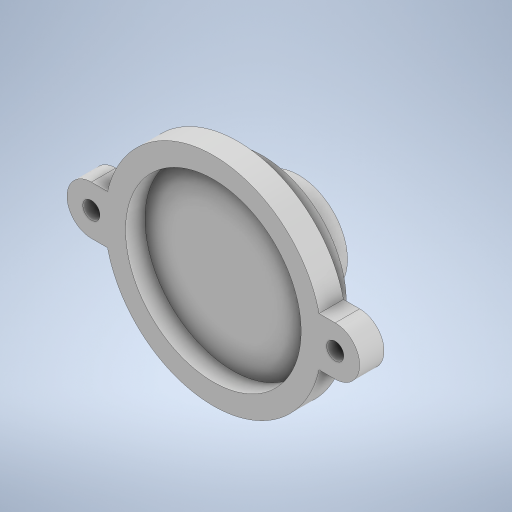
# Autodesk Inventor part: Prato do Amassador
Saved by Autodesk Inventor 2023 (Build 270158030, 158C)
## iProperties
Created: 2022-07-18
Part Number: Prato do Amassador
Material: Generic
Document SubType Name: Modeling
Designer: coqui
Density: 1 g/cm^3
Appearance: Default
Author: coqui
Autodesk Inventor part; units mm, degrees
ref_plane "YZ Plane" through (0, 0, 0) normal (1, 0, 0) x (0, 1, 0)
ref_plane "XZ Plane" through (0, 0, 0) normal (0, 1, 0) x (-1, 0, 0)
ref_plane "XY Plane" through (0, 0, 0) normal (0, 0, 1) x (1, 0, 0)
sketch "Sketch1" plane through (0, 0, 0) normal (0, 0, 1) x (1, 0, 0)
  arc A0 (50, -10) -> (50, 10) centre (50, 0) ccw
  arc A1 (-50, 10) -> (-50, -10) centre (-50, 0) ccw
  arc A2 (-43.3618, -10) -> (43.3618, -10) centre (0, 0) ccw
  arc A3 (43.3618, 10) -> (-43.3618, 10) centre (0, 0) ccw
  circle A4 centre (-50, 0) radius 3.5
  circle A5 centre (50, 0) radius 3.5
  line L0 (50, -10) -> (43.3618, -10)
  line L1 (-43.3618, -10) -> (-50, -10)
  line L2 (-50, 10) -> (-43.3618, 10)
  line L3 (43.3618, 10) -> (50, 10)
  dimension "d1" = 20
  dimension "d2" = 20
  dimension "d4" = 50
  dimension "d5" = 50
  dimension "d6" = 7
  dimension "d7" = 7
  constraints: 8 end point, 8 point on circle, 6 centre point, 6 tangent, 3 coincident
  measures "d1" diameter of A0
  measures "d2" diameter of A1
  measures "d4" distance of A0.centre point (0, 0)
  measures "d5" distance of point (0, 0) A1.centre
  measures "d6" diameter of A4
  measures "d7" diameter of A5
extrude "Extrusion1" add sketch "Sketch1" along normal blind 10
sketch "Sketch2" plane through (0, 0, 10) normal (0, 0, 1) x (1, 0, 0)
  circle A0 centre (0, 0) radius 36
  dimension "d10" = 72
  constraints: 1 centre point, 1 coincident
  measures "d10" diameter of A0
extrude "Extrusion2" cut sketch "Sketch2" against normal blind 8
sketch "Sketch3" plane through (0, 0, 0) normal (0, 0, -1) x (-1, 0, 0)
  circle A0 centre (0, 0) radius 34.5
  dimension "d13" = 69
  constraints: 1 centre point, 1 coincident
  measures "d13" diameter of A0
extrude "Extrusion3" add sketch "Sketch3" along normal blind 10
sketch "Sketch4" plane through (0, 0, -10) normal (0, 0, -1) x (-1, 0, 0)
  circle A0 centre (0, 0) radius 20
  dimension "d16" = 40
  constraints: 1 centre point, 1 coincident
  measures "d16" diameter of A0
extrude "Extrusion4" add sketch "Sketch4" along normal blind 15
sketch "Sketch6" plane through (0, 0, 0) normal (0, 1, 0) x (-1, 0, 0)
  line L0 (-34.5, 0) -> (-34.5, -10) projected
  line L1 (-34.5, 0) -> (-34, 0)
  line L2 (-34, 0) -> (-34, -3)
  line L3 (-34, -3) -> (-34.5, -3)
  line L4 (-34.5, -3) -> (-34.5, 0)
  line L5 (-34.5, -10) -> (34.5, -10) projected
  line L6 (-20, -10) -> (-20, -25) projected
  line L7 (-20, -10) -> (-19.5, -10)
  line L8 (-19.5, -10) -> (-19.5, -15)
  line L9 (-19.5, -15) -> (-20, -15)
  line L10 (-20, -15) -> (-20, -10)
  line L11 (0, 12.5498) -> (0, -27.5159) construction
  point P0 (0, 0)
  dimension "d19" = 0.5
  dimension "d20" = 3
  dimension "d21" = 7
  dimension "d22" = 0.5
  dimension "d23" = 5
  constraints: 18 end point, 4 parallel, 3 point on line, 2 horizontal, 2 perpendicular, 1 vertical
  measures "d19" distance of L2.end L3.end
  measures "d20" distance of L1.end L2.end
  measures "d21" distance between parallel lines of L5 L3
  measures "d22" distance of L8.end L9.end
  measures "d23" distance of L7.end L8.end
revolve "Revolution1" cut sketch "Sketch6" angle 360 about axis through (0, 0, 12.5498) along (0, 0, -1)
body "Solid1"
